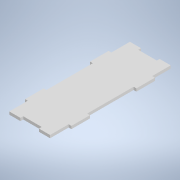
# Autodesk Inventor part: LongSide
Saved by Autodesk Inventor 2020.3 (Build 243373000, 373)
## iProperties
Created: 2020-08-22
Part Number: LongSide
Material: Generic
Document SubType Name: Modeling
Designer: Scott Hanson
Density: 1 g/cm^3
Appearance: Default
VerticalTab: 20.000 mm
Author: Scott Hanson
Autodesk Inventor part; units mm, degrees
ref_plane "YZ Plane" through (0, 0, 0) normal (1, 0, 0) x (0, 1, 0)
ref_plane "XZ Plane" through (0, 0, 0) normal (0, 1, 0) x (-1, 0, 0)
ref_plane "XY Plane" through (0, 0, 0) normal (0, 0, 1) x (1, 0, 0)
sketch "Sketch1" plane through (0, 0, 0) normal (0, 1, 0) x (-1, 0, 0)
  line L0 (0, 0) -> (-50, 0)
  line L1 (-50, 0) -> (-50, -130)
  line L2 (-50, -130) -> (0, -130)
  line L3 (0, -130) -> (0, 0)
  dimension "d0" = 130
  dimension "d1" = 50
  constraints: 8 end point, 2 parallel, 1 horizontal, 1 perpendicular
  measures "d0" distance of L2.end L0.start
  measures "d1" distance of L0.start L0.end
extrude "Base" add sketch "Sketch1" along normal blind 3
sketch "Sketch2" plane through (0, 3, 0) normal (0, 1, 0) x (1, 0, 0)
  line L0 (0, 0) -> (50, 0) projected
  line L1 (50, 130) -> (0, 130) projected
  line L2 (0, 0) -> (3, 0)
  line L3 (3, 130) -> (0, 130)
  line L4 (0, 130) -> (0, 0)
  line L5 (0, 130) -> (0, 0) projected
  line L6 (0, 0) -> (3, 0)
  line L7 (3, 0) -> (3, 20)
  line L8 (3, 20) -> (0, 20)
  line L9 (0, 20) -> (0, 0)
  line L10 (0, 130) -> (3, 130)
  line L11 (3, 130) -> (3, 110)
  line L12 (3, 110) -> (0, 110)
  line L13 (0, 110) -> (0, 130)
  line L14 (0, 40) -> (3, 40)
  line L15 (3, 40) -> (3, 90)
  line L16 (3, 90) -> (0, 90)
  line L17 (0, 90) -> (0, 40)
  line L18 (25, 0) -> (25, 130) construction
  line L19 (50, 0) -> (47, 0)
  line L20 (47, 130) -> (50, 130)
  line L21 (50, 130) -> (50, 0)
  line L22 (50, 130) -> (50, 0)
  line L23 (50, 0) -> (47, 0)
  line L24 (47, 0) -> (47, 20)
  line L25 (47, 20) -> (50, 20)
  line L26 (50, 20) -> (50, 0)
  line L27 (50, 130) -> (47, 130)
  line L28 (47, 130) -> (47, 110)
  line L29 (47, 110) -> (50, 110)
  line L30 (50, 110) -> (50, 130)
  line L31 (50, 40) -> (47, 40)
  line L32 (47, 40) -> (47, 90)
  line L33 (47, 90) -> (50, 90)
  line L34 (50, 90) -> (50, 40)
  line L35 (15, 0) -> (35, 0)
  line L36 (35, 0) -> (35, 3)
  line L37 (35, 3) -> (15, 3)
  line L38 (15, 3) -> (15, 0)
  line L39 (0, 65) -> (50, 65) construction
  line L40 (50, 0) -> (50, 130) projected
  line L41 (35, 130) -> (35, 127)
  line L42 (35, 127) -> (15, 127)
  line L43 (15, 127) -> (15, 130)
  point P0 (0, 20)
  point P1 (0, 110)
  point P2 (0, 130)
  point P3 (0, 90)
  point P4 (0, 40)
  point P5 (15, 130)
  dimension "d10" = 20
  dimension "d11" = 20
  dimension "d12" = 20
  dimension "d13" = 20
  dimension "d14" = 50
  dimension "d15" = 3
  dimension "VerticalTab" = 20
  dimension "d19" = 10
  dimension "d20" = 3
  constraints: 80 end point, 18 symmetric about line, 9 parallel, 8 point on line, 5 horizontal, 4 perpendicular, 3 midpoint, 2 other
  measures "d10" distance of L6.end L7.end
  measures "d11" distance of L10.end L11.end
  measures "d12" distance between parallel lines of L14 L8
  measures "d13" distance between parallel lines of L16 L12
  measures "d14" distance of L14.end L15.end
  measures "d15" distance of L7.end L8.end
  measures "VerticalTab" distance of L36.end L37.end
  measures "d19" distance from line of L18 L37.end
  measures "d20" distance of L35.end L36.end
extrude "Tabs" cut sketch "Sketch2" against normal through all contours L4 L8 L7 L0 | L38 L37 L36 L0 | L4 L16 L15 L14 | L24 L25 L21 L0 | L4 L1 L11 L12 | L31 L32 L33 L21 | L1 L41 L42 L43 | L29 L28 L1 L21
equation "\"d0\" = Length"
equation "\"d2\" = Thickness"
equation "\"d10\" = LengthTabOffset"
equation "\"d11\" = LengthTabOffset"
equation "\"d12\" = BaseTabWidth"
equation "\"d13\" = BaseTabWidth"
equation "\"d15\" = Thickness"
equation "\"d19\" = 0.5 * VerticalTab"
equation "\"d20\" = d15"
equation "\"Length\" = 130"
equation "\"Thickness\" = 3"
equation "\"LengthTabOffset\" = 20"
equation "\"BaseTabWidth\" = 20"
body "Solid1"
